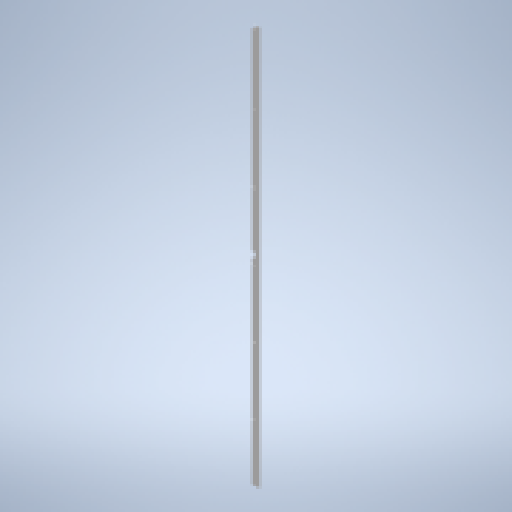
# Autodesk Inventor part: BSH 0442 stringer 42
Saved by Autodesk Inventor 2025 (Build 290162010, 162A)
## iProperties
Created: 2024-07-23
Part Number: BSH 0442 stringer 42
Material: 09g2s
Document SubType Name: Sheet Metal
Designer: DELL
Mass: 3894.87 g
Surface Area: 3485.79 cm^2
Volume: 496.162 cm^3
Density: 7.85 g/cm^3
Flat Pattern Width: 298 cm
Flat Pattern Length: 6.01073 cm
Flat Pattern Area: 1791.2 cm^2
Sheet Metal Rule: AISI304 3mm Die 32
Sheet Metal Width: 2980,000 mm
Sheet Metal Length: 60,107 mm
Sheet Metal Area: 179119,669 mm^2
Appearance: Default
Author: admin
Autodesk Inventor part; units mm, degrees
ref_plane "YZ Plane" through (0, 0, 0) normal (1, 0, 0) x (0, 1, 0)
ref_plane "XZ Plane" through (0, 0, 0) normal (0, 1, 0) x (-1, 0, 0)
ref_plane "XY Plane" through (0, 0, 0) normal (0, 0, 1) x (1, 0, 0)
sketch "Sketch6" plane through (0, 0, 0) normal (0, 1, 0) x (-1, 0, 0)
  line L0 (0, 0) -> (-60.1073, 0)
  line L1 (-60.1073, 0) -> (-60.1073, 2980)
  line L2 (-60.1073, 2980) -> (0, 2980)
  line L3 (0, 2980) -> (0, 0)
  dimension "d26" = 60.1073
  dimension "d27" = 2980
  measures "d26" distance of L1.end L2.end
  measures "d27" distance of L0.end L1.end
extrude "Plate4" add sketch "Sketch6" along normal blind 3
sketch "Sketch9" plane through (0, 3, 0) normal (0, 1, 0) x (1, 0, 0)
  line L0 (0, -2980) -> (0, 0) projected
  line L1 (60.1073, -2980) -> (0, -2980) projected
  line L2 (60.1073, 0) -> (60.1073, -2980) projected
  line L3 (0, 0) -> (60.1073, 0) projected
  line L4 (25, -210) -> (10, -210) construction
  line L5 (10, -210) -> (10, -10) construction
  line L6 (10, -10) -> (25, -10) construction
  line L7 (25, -10) -> (25, -210) construction
  dimension "d44" = 200
  dimension "d45" = 15
  dimension "d46" = 10
  dimension "d47" = 10
  constraints: 1 vertical, 2 other
  measures "d44" distance of L4.end L5.end
  measures "d45" distance between parallel lines of L5 L7
  measures "d46" distance from line of L3 L5.end
  measures "d47" distance between parallel lines of L5 L0
sketch "Sketch7" plane through (0, 0, 0) normal (0, -1, 0) x (1, 0, 0)
  line L0 (0, 2980) -> (60.1073, 2980) projected
  line L1 (0, 0) -> (0, 2980) projected
  line L2 (60.1073, 0) -> (0, 0) projected
  line L3 (60.1073, 2980) -> (60.1073, 0) projected
  line L4 (0, 430.2) -> (31.0536, 430.2)
  line L5 (31.0536, 430.2) -> (31.0536, 427)
  line L6 (31.0536, 427) -> (0, 427)
  line L7 (0, 427) -> (0, 430.2)
  point P0 (0, 427)
  point P1 (0, 200)
  point P2 (46.4173, 200)
  point P3 (0, 427)
  dimension "d29" = 31.0536
  dimension "d30" = 3.2
  dimension "d31" = 427
  constraints: 8 end point, 2 parallel, 1 horizontal, 1 perpendicular, 1 point on line
  measures "d29" distance of L5.end L6.end
  measures "d30" distance of L4.end L5.end
  measures "d31" distance between parallel lines of L2 L6
extrude "Extrusion2" cut sketch "Sketch7" against normal through all contours L4 L5 L6 L1
pattern_linear "Rectangular Pattern1" count 5 spacing 500 along (0, 0, 1) of "Extrusion2"
sketch "Sketch8" plane through (0, 0, 0) normal (0, -1, 0) x (1, 0, 0)
  line L0 (0, 1930.2) -> (0, 2427) projected
  line L1 (0, 430.2) -> (31.0536, 430.2) projected
  line L2 (31.0536, 430.2) -> (31.0536, 427) projected
  line L3 (31.0536, 427) -> (0, 427) projected
  line L4 (0, 0) -> (0, 427) projected
  line L5 (60.1073, 0) -> (0, 0) projected
  line L6 (60.1073, 2980) -> (60.1073, 0) projected
  line L7 (0, 2980) -> (60.1073, 2980) projected
  circle A0 centre (0, 1490) radius 25
  line L8 (0, 1930.2) -> (31.0536, 1930.2) projected
  line L9 (31.0536, 1930.2) -> (31.0536, 1927) projected
  line L10 (31.0536, 1927) -> (0, 1927) projected
  line L11 (0, 1430.2) -> (0, 1927) projected
  line L12 (0, 1430.2) -> (31.0536, 1430.2) projected
  line L13 (31.0536, 1430.2) -> (31.0536, 1427) projected
  line L14 (31.0536, 1427) -> (0, 1427) projected
  line L15 (0, 930.2) -> (0, 1427) projected
  line L16 (0, 930.2) -> (31.0536, 930.2) projected
  line L17 (31.0536, 930.2) -> (31.0536, 927) projected
  line L18 (31.0536, 927) -> (0, 927) projected
  line L19 (0, 430.2) -> (0, 927) projected
  line L20 (0, 2430.2) -> (31.0536, 2430.2) projected
  line L21 (31.0536, 2430.2) -> (31.0536, 2427) projected
  line L22 (31.0536, 2427) -> (0, 2427) projected
  line L23 (0, 2430.2) -> (0, 2980) projected
  dimension "d37" = 50
  dimension "d38" = 1490
  constraints: 1 centre point
  measures "d37" diameter of A0
  measures "d38" distance from line of A0.centre L5
extrude "Extrusion3" cut sketch "Sketch8" against normal through all contours L11 A0 | A0 L11
pattern_linear "Rectangular Pattern2" count 3 spacing 1480 along (0, 0, 1) of "Extrusion3" first direction both ways yes
mark "Mark1"
chamfer "Corner Chamfer1" distance 6 angle 45 1 edges at (60.1073, 1.5, 2980)
equation "\"d26\" = Stringer4_deep"
equation "\"d28\" = Thickness"
equation "\"BendReliefWidth\" = Thickness"
equation "\"BendReliefDepth\" = 0.5 * Thickness"
equation "\"CornerReliefSize\" = 4 * Thickness"
equation "\"MinimumRemnant\" = 2 * Thickness"
equation "\"TransitionRadius\" = BendRadius"
equation "\"JacobiRadiusSize\" = BendRadius"
equation "\"GapSize\" = Thickness"
equation "\"Stringer4_deep\" = 60.107271"
equation "\"Thickness\" = 3"
equation "\"BendRadius\" = 5"
body "Solid2"
